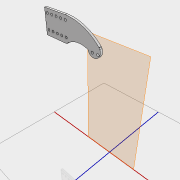
# Autodesk Inventor part: ЛЦМК000002.00.00.00.00.20 Платформа экрана
Saved by Autodesk Inventor 2021.2 (Build 252289000, 289)
## iProperties
Created: 2025-11-11
Part Number: ЛЦМК000002.00.00.00.00.20 Платформа экрана
Material: Типовые
Document SubType Name: Modeling
Designer: Захаров
Density: 1 g/cm^3
Appearance: По умолчанию
Author: Захаров
Autodesk Inventor part; units mm, degrees
ref_plane "YZ Plane" through (0, 0, 0) normal (1, 0, 0) x (0, 1, 0)
ref_plane "XZ Plane" through (0, 0, 0) normal (0, 1, 0) x (-1, 0, 0)
ref_plane "XY Plane" through (0, 0, 0) normal (0, 0, 1) x (1, 0, 0)
ref_plane "РабПлоскость1" through (0, 0, 0) normal (0, 0, 1) x (1, 0, 0)
sketch "Эскиз1" plane through (0, 0, 0) normal (0, 0, 1) x (1, 0, 0)
  line L0 (-3.6964, 47.257) -> (-93.6964, 47.257)
  line L1 (-93.6964, 47.257) -> (-93.6964, 77.257)
  line L2 (-93.6964, 77.257) -> (-3.6964, 77.257)
  line L3 (-3.6964, 77.257) -> (-3.6964, 47.257)
  circle A0 centre (-25.0996, 50.4451) radius 1.5 projected
  circle A1 centre (-61.7063, 54.0675) radius 1.5
  circle A2 centre (-68.7063, 54.0675) radius 1.5
  circle A3 centre (-75.7063, 54.0675) radius 1.5
  circle A4 centre (-82.7063, 54.0675) radius 1.5
  circle A5 centre (-89.7063, 54.0675) radius 1.5
  circle A6 centre (-61.7063, 72.0675) radius 1.5
  circle A7 centre (-68.7063, 72.0675) radius 1.5
  circle A8 centre (-75.7063, 72.0675) radius 1.5
  circle A9 centre (-82.7063, 72.0675) radius 1.5
  circle A10 centre (-89.7063, 72.0675) radius 1.5
  circle A11 centre (-5.0903, 22.9004) radius 1.5 projected
  circle A12 centre (-13.6314, 40.9849) radius 1.5 projected
  circle A13 centre (7.7213, -4.2264) radius 1.5 projected
  circle A14 centre (-0.8198, 13.8581) radius 1.5 projected
  circle A15 centre (3.4507, 4.8159) radius 1.5 projected
  circle A16 centre (11.9918, -13.2686) radius 1.5 projected
  circle A17 centre (-9.3609, 31.9427) radius 1.5 projected
  circle A18 centre (16.2623, -22.3109) radius 1.5 projected
  circle A19 centre (-9.4594, 1.6491) radius 1.5 projected
  circle A20 centre (-3.3563, -17.3969) radius 1.5 projected
  circle A21 centre (-18.6141, 30.2182) radius 1.5 projected
  circle A22 centre (-12.511, 11.1722) radius 1.5 projected
  circle A23 centre (-15.5626, 20.6952) radius 1.5 projected
  circle A24 centre (-21.6657, 39.7412) radius 1.5 projected
  circle A25 centre (-6.4079, -7.8739) radius 1.5 projected
  circle A26 centre (-0.3048, -26.9199) radius 1.5 projected
  arc A27 (1.815, -50.7724) -> (29.663, -39.7893) centre (16.0996, -46.1951) ccw projected
  line L4 (29.663, -39.7893) -> (-15.8657, 56.6115) projected
  arc A28 (-15.8657, 56.6115) -> (-16.7091, 58.0078) centre (-23.0996, 53.1951) ccw projected
  arc A29 (-16.7091, 58.0078) -> (-17.3202, 58.7267) centre (-18.0996, 57.4451) ccw projected
  arc A30 (-17.3202, 58.7267) -> (-30.8744, 51.3105) centre (-23.0996, 53.1951) ccw projected
  arc A31 (-30.6007, 50.3877) -> (-30.8744, 51.3105) centre (-32.0996, 50.4451) ccw projected
  line L5 (-30.6007, 50.3877) -> (1.815, -50.7724) projected
  circle A32 centre (25.6634, -44.4774) radius 1.5 projected
  circle A33 centre (5.6634, -44.4774) radius 1.5 projected
  circle A34 centre (-25.0996, 50.4451) radius 1.5 projected
  arc A35 (-16.9566, 58.4165) -> (-61.7063, 77.257) centre (-63.0326, 11.5423) ccw
  arc A36 (-30.8744, 51.3105) -> (-61.7063, 47.257) centre (-43.024, 24.4392) ccw
  arc A37 (-30.6007, 50.3877) -> (-15.918, 56.7222) centre (-23.1518, 53.3058) ccw
  arc A38 (-16.5996, 50.4451) -> (-19.5996, 50.4451) centre (-18.0996, 50.4451) ccw projected
  arc A39 (-18.1711, 45.521) -> (-16.5996, 50.4451) centre (-25.0996, 50.4451) ccw projected
  arc A40 (-20.6164, 47.2589) -> (-18.1711, 45.521) centre (-19.3937, 46.39) ccw projected
  arc A41 (-20.6164, 47.2589) -> (-19.5996, 50.4451) centre (-25.0996, 50.4451) ccw projected
  arc A42 (-16.5996, 50.4451) -> (-19.5996, 50.4451) centre (-18.0996, 50.4451) ccw projected
  point P0 (0, 0)
  point P1 (-15.8921, 56.6667)
  dimension "d0" = 90
  dimension "d1" = 30
  dimension "d2" = 3
  dimension "d5" = 7
  dimension "d8" = 18
  constraints: 13 centre point, 8 end point, 7 point on circle, 3 point on line, 2 horizontal, 2 parallel, 1 equal radius, 1 perpendicular, 1 tangent, 1 vertical, 18 other
  measures "d0" distance of L1.end L2.end
  measures "d1" distance of L0.end L1.end
  measures "d2" diameter of A1
  measures "d5" distance of A1.centre A2.centre
  measures "d8" distance of A1.centre A6.centre
extrude "Выдавливание1" add sketch "Эскиз1" along normal blind 2 contours L0 L1 L2 A35 A29 A30 A36 | A30 A29 A35 A28 A37 A39 A38 A41 L0 A31 | L0 A40 A37 | A41 A38 A39 A37 L0 | L0 A37 A40
sketch "Эскиз2" plane through (0, 0, 2) normal (0, 0, 1) x (1, 0, 0)
  line L0 (-83.9909, 70.7175) -> (-91.1909, 70.7175) projected
  line L1 (-91.1909, 70.7175) -> (-91.1909, 74.5675) projected
  line L2 (-91.1909, 74.5675) -> (-50.1909, 74.5675) projected
  line L3 (-50.1909, 74.5675) -> (-50.1909, 72.0675) projected
  line L4 (-50.1909, 72.0675) -> (-58.3909, 72.0675) projected
  line L5 (-58.3909, 72.0675) -> (-58.3909, 54.0675) projected
  line L6 (-58.3909, 54.0675) -> (-50.1909, 54.0675) projected
  line L7 (-50.1909, 54.0675) -> (-50.1909, 51.3675) projected
  line L8 (-50.1909, 51.3675) -> (-91.1909, 51.3675) projected
  line L9 (-91.1909, 51.3675) -> (-91.1909, 55.2175) projected
  line L10 (-91.1909, 55.2175) -> (-83.9909, 55.2175) projected
  line L11 (-83.9909, 55.2175) -> (-83.9909, 70.7175) projected
  circle A0 centre (-82.7063, 72.0675) radius 1.5 projected
  circle A1 centre (-61.7063, 54.0675) radius 1.5 projected
  circle A2 centre (-61.7063, 72.0675) radius 1.5 projected
  circle A3 centre (-82.7063, 54.0675) radius 1.5 projected
  arc A4 (-15.8921, 56.6667) -> (-16.7091, 58.0078) centre (-23.0996, 53.1951) ccw projected
  arc A5 (-16.7091, 58.0078) -> (-16.9566, 58.4165) centre (-18.0996, 57.4451) ccw projected
  arc A6 (-16.9566, 58.4165) -> (-61.7063, 77.257) centre (-63.0326, 11.5423) ccw projected
  line L12 (-61.7063, 77.257) -> (-93.6964, 77.257) projected
  line L13 (-93.6964, 77.257) -> (-93.6964, 47.257) projected
  line L14 (-93.6964, 47.257) -> (-61.7063, 47.257) projected
  arc A7 (-30.8744, 51.3105) -> (-61.7063, 47.257) centre (-43.024, 24.4392) ccw projected
  arc A8 (-30.6007, 50.3877) -> (-30.8744, 51.3105) centre (-32.0996, 50.4451) ccw projected
  arc A9 (-30.6007, 50.3877) -> (-15.8921, 56.6667) centre (-23.1518, 53.3058) ccw projected
  circle A10 centre (-61.7063, 54.0675) radius 1.5 projected
  circle A11 centre (-61.7063, 72.0675) radius 1.5 projected
  circle A12 centre (-82.7063, 72.0675) radius 1.5 projected
  circle A13 centre (-68.7063, 72.0675) radius 1.5 projected
  circle A14 centre (-68.7063, 54.0675) radius 1.5 projected
  circle A15 centre (-75.7063, 54.0675) radius 1.5 projected
  circle A16 centre (-82.7063, 54.0675) radius 1.5 projected
  circle A17 centre (-89.7063, 54.0675) radius 1.5 projected
  circle A18 centre (-75.7063, 72.0675) radius 1.5 projected
  circle A19 centre (-89.7063, 72.0675) radius 1.5 projected
  circle A20 centre (-25.0996, 50.4451) radius 1.5 projected
  line L15 (-93.6964, 77.257) -> (-93.6964, 47.257) projected
  line L16 (-91.1909, 51.3675) -> (-93.6964, 51.3675)
  line L17 (-93.6964, 51.3675) -> (-93.6964, 74.5675)
  line L18 (-93.6964, 74.5675) -> (-91.1909, 74.5675)
  line L19 (-91.1909, 74.5675) -> (-91.1909, 51.3675)
  line L20 (-50.1909, 74.5675) -> (-44.3775, 74.5675)
  point P0 (0, 0)
  point P1 (-91.1909, 54.2816)
  point P2 (-91.1909, 53.8534)
  point P3 (-91.1909, 72.2816)
  point P4 (-91.1909, 71.8534)
  point P5 (-55.0469, 51.3675)
  constraints: 10 end point, 2 horizontal, 2 parallel, 1 perpendicular, 1 point on circle, 1 point on line
extrude "Выдавливание2" cut sketch "Эскиз2" against normal blind 3 contours A19 L1 | L18 L13 L12 A6 L20 L2 | L9 A17 | L8 A7 L14 L13 L16
